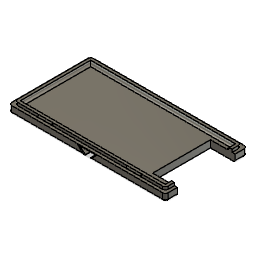
ROC_rev_C_screw_terminal_bottom (Autodesk Fusion 360 design; units mm, degrees)
Autodesk Fusion 360 part; units mm, degrees
sketch "Sketch13" plane through (0, 16, -2.5) normal (0, -1, 0) x (1, 0, 0)
  line L0 (26.9, -45.4) -> (26.9, -60.4)
  arc A0 (24.9, -62.4) -> (26.9, -60.4) centre (24.9, -60.4) ccw
  line L1 (24.9, -62.4) -> (-24.9, -62.4)
  arc A1 (-26.9, -60.4) -> (-24.9, -62.4) centre (-24.9, -60.4) ccw
  line L2 (-26.9, -60.4) -> (-26.9, -45.4)
  line L3 (-26.9, -45.4) -> (-26.9, -35.4)
  line L4 (-26.9, -35.4) -> (-26.9, 17.4)
  line L5 (-26.9, 17.4) -> (-26.9, 27.4)
  line L6 (-26.9, 27.4) -> (-26.9, 42.4)
  arc A2 (-24.9, 44.4) -> (-26.9, 42.4) centre (-24.9, 42.4) ccw
  line L7 (-24.9, 44.4) -> (24.9, 44.4)
  arc A3 (26.9, 42.4) -> (24.9, 44.4) centre (24.9, 42.4) ccw
  line L8 (26.9, 42.4) -> (26.9, 27.4)
  line L9 (26.9, 27.4) -> (26.9, 17.4)
  line L10 (26.9, 17.4) -> (26.9, -35.4)
  line L11 (26.9, -35.4) -> (26.9, -45.4)
  arc A4 (29, 44.5) -> (27, 46.5) centre (27, 44.5) ccw
  line L12 (27, 46.5) -> (-27, 46.5)
  arc A5 (-27, 46.5) -> (-29, 44.5) centre (-27, 44.5) ccw
  line L13 (-29, 44.5) -> (-29, -62.5)
  arc A6 (-29, -62.5) -> (-27, -64.5) centre (-27, -62.5) ccw
  line L14 (-27, -64.5) -> (27, -64.5)
  arc A7 (27, -64.5) -> (29, -62.5) centre (27, -62.5) ccw
  line L15 (29, -62.5) -> (29, 44.5)
  line L16 (-26.9, -35.4) -> (-29, -35.4)
  line L17 (-29, -35.4) -> (-29, -45.4)
  line L18 (-29, -45.4) -> (-26.9, -45.4)
  line L19 (-26.9, -45.4) -> (-26.9, -35.4)
  line L20 (-26.9, 27.4) -> (-29, 27.4)
  line L21 (-29, 27.4) -> (-29, 17.4)
  line L22 (-29, 17.4) -> (-26.9, 17.4)
  line L23 (-26.9, 17.4) -> (-26.9, 27.4)
  line L24 (26.9, 27.4) -> (29, 27.4)
  line L25 (29, 27.4) -> (29, 17.4)
  line L26 (29, 17.4) -> (26.9, 17.4)
  line L27 (26.9, 17.4) -> (26.9, 27.4)
  line L28 (26.9, -35.4) -> (29, -35.4)
  line L29 (29, -35.4) -> (29, -45.4)
  line L30 (29, -45.4) -> (26.9, -45.4)
  line L31 (26.9, -45.4) -> (26.9, -35.4)
  dimension "d1" = 10
  dimension "d2" = 2.1
  dimension "d3" = 10
  dimension "d4" = 10
  dimension "d5" = 10
  constraint horizontal L16
  constraint vertical L17
  constraint horizontal L18
  constraint vertical L19
  constraint coincident L3.end L4.start
  constraint horizontal L20
  constraint vertical L21
  constraint horizontal L22
  constraint vertical L23
  constraint coincident L5.end L6.start
  constraint horizontal L24
  constraint vertical L25
  constraint horizontal L26
  constraint vertical L27
  constraint coincident L8.end L9.start
  constraint horizontal L28
  constraint vertical L29
  constraint horizontal L30
  constraint vertical L31
  constraint coincident L10.end L11.start
  measures "d1" distance of L3.end L2.end
  measures "d2" distance of L5.end L20.end
  measures "d3" distance of L5.end L4.end
  measures "d4" distance of L8.end L9.end
  measures "d5" distance of L10.end L0.start
sketch "Sketch2" plane through (0, 0, 0) normal (0, 1, 0) x (1, 0, 0)
  line L0 (53.5, -29) -> (-53.5, -29)
  line L1 (-55.5, -27) -> (-55.5, 27)
  line L2 (-53.5, 29) -> (53.5, 29)
  line L3 (55.5, 27) -> (55.5, -27)
  line L4 (55.5, -29) -> (-55.5, 29) construction
  line L5 (-55.5, -29) -> (55.5, 29) construction
  arc A0 (-53.5, 29) -> (-55.5, 27) centre (-53.5, 27) ccw
  arc A1 (55.5, 27) -> (53.5, 29) centre (53.5, 27) ccw
  arc A2 (53.5, -29) -> (55.5, -27) centre (53.5, -27) ccw
  arc A3 (-55.5, -27) -> (-53.5, -29) centre (-53.5, -27) ccw
  dimension "d255" = 111
  dimension "d256" = 58
  dimension "d257" = 2
  dimension "d265" = 0
  dimension "d266" = 0
  dimension "d267" = 0
  dimension "d268" = 0
  dimension "d442" = 0
  dimension "d443" = 0
  dimension "d444" = 0
  dimension "d445" = 0
  dimension "d460" = 0
  dimension "d461" = 0
  dimension "d462" = 0
  dimension "d463" = 0
  constraint perpendicular L0 L1
  constraint parallel L0 L2
  constraint parallel L1 L3
  constraint horizontal L0
  constraint coincident L4 origin
  constraint coincident L5 origin
  constraint coincident L4.end L1
  constraint coincident L4.end L2
  constraint tangent L1 A0
  constraint tangent L2 A0
  constraint coincident L5.end L2
  constraint coincident L5.end L3
  constraint tangent L2 A1
  constraint tangent L3 A1
  constraint equal A0 A1
  constraint coincident L4.start L3
  constraint coincident L4.start L0
  constraint tangent L3 A2
  constraint tangent L0 A2
  constraint equal A0 A2
  constraint coincident L5.start L0
  constraint coincident L5.start L1
  constraint tangent L0 A3
  constraint tangent L1 A3
  constraint equal A0 A3
  measures "d255" distance of L4.end L5.end
  measures "d256" distance of L5.start L4.end
  measures "d257" radius of A0
extrude "Extrude1" add sketch "Sketch2" along normal blind 5
sketch "Sketch3" plane through (0, 5, 0) normal (0, 1, 0) x (-1, 0, 0)
  arc A0 (53.5, -29) -> (55.5, -27) centre (53.5, -27) ccw
  line L0 (55.5, -27) -> (55.5, 27)
  arc A1 (55.5, 27) -> (53.5, 29) centre (53.5, 27) ccw
  line L1 (53.5, 29) -> (-53.5, 29)
  arc A2 (-53.5, 29) -> (-55.5, 27) centre (-53.5, 27) ccw
  line L2 (-55.5, 27) -> (-55.5, -27)
  arc A3 (-55.5, -27) -> (-53.5, -29) centre (-53.5, -27) ccw
  line L3 (-53.5, -29) -> (53.5, -29)
  line L4 (53.4, -24.9) -> (53.4, 24.9)
  line L5 (51.4, 26.9) -> (-51.4, 26.9)
  line L6 (-53.4, 24.9) -> (-53.4, -24.9)
  line L7 (-51.4, -26.9) -> (51.4, -26.9)
  arc A4 (51.4, -26.9) -> (53.4, -24.9) centre (51.4, -24.9) ccw
  arc A5 (-53.4, -24.9) -> (-51.4, -26.9) centre (-51.4, -24.9) ccw
  arc A6 (-51.4, 26.9) -> (-53.4, 24.9) centre (-51.4, 24.9) ccw
  arc A7 (53.4, 24.9) -> (51.4, 26.9) centre (51.4, 24.9) ccw
  line L8 (-51.4, 24.9) -> (-51.4, -24.9)
  line L9 (-51.4, -24.9) -> (51.4, -24.9)
  line L10 (51.4, -24.9) -> (51.4, 24.9)
  line L11 (51.4, 24.9) -> (-51.4, 24.9)
  dimension "d261" = 2
  dimension "d262" = -2
  dimension "d277" = 2.1
  dimension "d278" = 2.1
  dimension "d279" = 2.1
  dimension "d280" = 2.1
  constraint parallel L0 L4
  constraint parallel L1 L5
  constraint parallel L2 L6
  constraint parallel L3 L7
  constraint tangent L4 A4
  constraint tangent L7 A4
  constraint tangent L7 A5
  constraint tangent L6 A5
  constraint equal A4 A5
  constraint tangent L5 A6
  constraint tangent L6 A6
  constraint equal A4 A6
  constraint tangent L5 A7
  constraint tangent L4 A7
  constraint equal A4 A7
  measures "d261" radius of A4
  measures "d277" distance of L3 L7
  measures "d278" distance of L0 L4
  measures "d279" distance of L1 L5
  measures "d280" distance of L2 L6
extrude "Extrude2" add sketch "Sketch3" along normal blind 2 contours L4 L5 L6 L7 A4 A5 A6 A7
sketch "Sketch4" plane through (0, 0, 26.9) normal (0, 0, 1) x (1, 0, 0)
  line L0 (-51.4, 5) -> (51.4, 5)
  line L1 (51.4, 5) -> (51.4, 7)
  line L2 (51.4, 7) -> (-51.4, 7)
  line L3 (-51.4, 7) -> (-51.4, 5)
  line L4 (36.4, 7) -> (26.4, 7)
  line L5 (26.4, 7) -> (26.4, 2)
  line L6 (26.4, 2) -> (36.4, 2)
  line L7 (36.4, 2) -> (36.4, 7)
  line L8 (-26.4, 7) -> (-36.4, 7)
  line L9 (-36.4, 7) -> (-36.4, 2)
  line L10 (-36.4, 2) -> (-26.4, 2)
  line L11 (-26.4, 2) -> (-26.4, 7)
  dimension "d289" = 10
  dimension "d290" = 10
  dimension "d291" = 15
  dimension "d292" = 15
  constraint horizontal L4
  constraint vertical L5
  constraint horizontal L6
  constraint vertical L7
  constraint coincident L2 L4.start
  constraint horizontal L8
  constraint vertical L9
  constraint horizontal L10
  constraint vertical L11
  constraint coincident L2 L8.start
  measures "d289" distance of L4.start L4.end
  measures "d290" distance of L8.start L8.end
  measures "d291" distance of L3 L9
  measures "d292" distance of L1 L7
extrude "Extrude3" add sketch "Sketch4" along normal blind 1 contours L0 L2 L8 L9 L11 | L0 L2 L4 L5 L7
sketch "Sketch5" plane through (-36.4, 0, 0) normal (-1, 0, 0) x (0, 0, 1)
  line L0 (26.9, 7) -> (26.9, 5)
  line L1 (26.9, 5) -> (27.9, 5)
  line L2 (27.9, 5) -> (27.9, 7)
  line L3 (27.9, 7) -> (26.9, 7)
  line L4 (26.9, 7) -> (27.9, 6)
  line L5 (26.9, 5) -> (27.9, 6)
  constraint coincident L0.start L3.end
  constraint midpoint L2 L4.end
  constraint coincident L0.end L1.start
extrude "Extrude4" cut sketch "Sketch5" against normal up to surface (72.8 mm away) contours L2 L3 L4 | L1 L2 L5
sketch "Sketch6" plane through (0, 0, -26.9) normal (0, 0, -1) x (-1, 0, 0)
  line L0 (-51.4, 5) -> (51.4, 5)
  line L1 (51.4, 5) -> (51.4, 7)
  line L2 (51.4, 7) -> (-51.4, 7)
  line L3 (-51.4, 7) -> (-51.4, 5)
  line L4 (36.4, 7) -> (26.4, 7)
  line L5 (26.4, 7) -> (26.4, 2)
  line L6 (26.4, 2) -> (36.4, 2)
  line L7 (36.4, 2) -> (36.4, 7)
  line L8 (-26.4, 7) -> (-36.4, 7)
  line L9 (-36.4, 7) -> (-36.4, 2)
  line L10 (-36.4, 2) -> (-26.4, 2)
  line L11 (-26.4, 2) -> (-26.4, 7)
  dimension "d297" = 10
  dimension "d298" = 10
  dimension "d299" = 15
  dimension "d300" = 15
  constraint horizontal L4
  constraint vertical L5
  constraint horizontal L6
  constraint vertical L7
  constraint coincident L2 L4.start
  constraint horizontal L8
  constraint vertical L9
  constraint horizontal L10
  constraint vertical L11
  constraint coincident L2 L8.start
  measures "d297" distance of L4.start L4.end
  measures "d298" distance of L8.start L8.end
  measures "d299" distance of L1 L7
  measures "d300" distance of L3 L9
extrude "Extrude5" add sketch "Sketch6" along normal blind 1 contours L0 L2 L8 L9 L11 | L0 L2 L4 L5 L7
sketch "Sketch7" plane through (36.4, 0, 0) normal (1, 0, 0) x (0, 0, -1)
  line L0 (26.9, 7) -> (26.9, 5)
  line L1 (26.9, 5) -> (27.9, 5)
  line L2 (27.9, 5) -> (27.9, 7)
  line L3 (27.9, 7) -> (26.9, 7)
  line L4 (26.9, 7) -> (27.9, 6)
  line L5 (27.9, 6) -> (26.9, 5)
  constraint coincident L0.start L3.end
  constraint midpoint L2 L4.end
  constraint coincident L0.end L1.start
extrude "Extrude6" cut sketch "Sketch7" against normal up to surface (72.8 mm away) contours L2 L3 L4 | L1 L2 L5
extrude "Extrude7" cut sketch "Sketch13" against normal blind 1 contours L11 L15 L28 L29 L30 L31 | L9 L15 L24 L25 L26 L27 | L3 L13 L16 L17 L18 L19 | L5 L13 L20 L21 L22 L23
chamfer "Chamfer1" [no effect]
fillet "Fillet1" radius 0.1 4 edges at (-31.4, 6, 27.9) (31.4, 6, 27.9) (-31.4, 6, -27.9) (31.4, 6, -27.9)
fillet "Fillet2" radius 1 8 edges at (-54.9142, 0, 28.4142) (-55.5, 0, 0) (-54.9142, 0, -28.4142) (0, 0, -29) (54.9142, 0, -28.4142) (55.5, 0, 0) (54.9142, 0, 28.4142) (0, 0, 29)
sketch "Sketch11" plane through (0, 5, 0) normal (0, 1, 0) x (-1, 0, 0)
  line L0 (-36.4, -26.9) -> (-51.4, -26.9)
  arc A0 (-53.4, -24.9) -> (-51.4, -26.9) centre (-51.4, -24.9) ccw
  line L1 (-53.4, -24.9) -> (-53.4, 24.9)
  arc A1 (-51.4, 26.9) -> (-53.4, 24.9) centre (-51.4, 24.9) ccw
  line L2 (-51.4, 26.9) -> (-36.4, 26.9)
  line L3 (53.5, 29) -> (-53.5, 29)
  arc A2 (-53.5, 29) -> (-55.5, 27) centre (-53.5, 27) ccw
  line L4 (-55.5, 27) -> (-55.5, -27)
  arc A3 (-55.5, -27) -> (-53.5, -29) centre (-53.5, -27) ccw
  line L5 (-53.5, -29) -> (53.5, -29)
  line L6 (-73, 20.5) -> (-38, 20.5)
  line L7 (-38, 20.5) -> (-38, -20.5)
  line L8 (-38, -20.5) -> (-73, -20.5)
  line L9 (-73, -20.5) -> (-73, 20.5)
  line L10 (-73, 20.5) -> (-38, -20.5) construction
  line L11 (-38, 20.5) -> (-73, -20.5) construction
  line L12 (-36.4, 26.9) -> (-26.4, 26.9)
  line L13 (-26.4, 26.9) -> (26.4, 26.9)
  line L14 (26.4, 26.9) -> (36.4, 26.9)
  line L15 (36.4, 26.9) -> (51.4, 26.9)
  arc A4 (53.4, 24.9) -> (51.4, 26.9) centre (51.4, 24.9) ccw
  line L16 (53.4, 24.9) -> (53.4, -24.9)
  arc A5 (51.4, -26.9) -> (53.4, -24.9) centre (51.4, -24.9) ccw
  line L17 (51.4, -26.9) -> (36.4, -26.9)
  line L18 (36.4, -26.9) -> (26.4, -26.9)
  line L19 (26.4, -26.9) -> (-26.4, -26.9)
  line L20 (-26.4, -26.9) -> (-36.4, -26.9)
  arc A6 (53.5, -29) -> (55.5, -27) centre (53.5, -27) ccw
  line L21 (55.5, -27) -> (55.5, 27)
  arc A7 (55.5, 27) -> (53.5, 29) centre (53.5, 27) ccw
  point P0 (-55.5, 0)
  dimension "d424" = 35
  dimension "d425" = 41
  constraint horizontal L6
  constraint perpendicular L6 L7
  constraint parallel L6 L8
  constraint parallel L7 L9
  constraint coincident L10 P0
  constraint coincident L11 P0
  constraint midpoint L4 P0
  measures "d424" distance of L6.start L6.end
  measures "d425" distance of L6.start L8.end
extrude "Extrude12" cut sketch "Sketch11" along normal mid plane 14 contours L1 L4 L6 L8 | L1 L6 L7 L8
sketch "Sketch12" plane through (0, 0, 29) normal (0, 0, 1) x (1, 0, 0)
  line L0 (-53.5, 1) -> (53.5, 1)
  line L1 (53.5, 1) -> (53.5, 5)
  line L2 (53.5, 5) -> (-53.5, 5)
  line L3 (-53.5, 5) -> (-53.5, 1)
  line L4 (-5.5, 4) -> (5.5, 4)
  line L5 (5.5, 4) -> (5.5, -4)
  line L6 (5.5, -4) -> (-5.5, -4)
  line L7 (-5.5, -4) -> (-5.5, 4)
  line L8 (-5.5, 4) -> (5.5, -4) construction
  line L9 (5.5, 4) -> (-5.5, -4) construction
  line L10 (5.5, 0) -> (-5.5, 0)
  line L11 (5.5, 4) -> (11.438, 4) construction
  line L12 (-5.5, 4) -> (-1.5, 0)
  line L13 (-5.5, 4) -> (1, 4) construction
  line L14 (5.5, 4) -> (1.5, 0)
  line L15 (0.8684, -0.6316) -> (0.7116, -0.7884)
  dimension "d428" = 11
  dimension "d429" = 8
  dimension "d432" = 135
  dimension "d433" = 45
  constraint horizontal L4
  constraint perpendicular L4 L5
  constraint parallel L4 L6
  constraint parallel L5 L7
  constraint coincident L8 origin
  constraint coincident L9 origin
  constraint midpoint L5 L10.start
  constraint midpoint L7 L10.end
  constraint horizontal L11
  constraint horizontal L13
  constraint coincident L10 L14.end
  constraint coincident L8 L15.start
  constraint collinear L14 L15
  constraint coincident L10 L12.end
  measures "d428" distance of L5.end L6.end
  measures "d429" distance of L4.end L5.end
  measures "d432" angle of L11 L14
  measures "d433" angle of L12 L13
extrude "Extrude13" cut sketch "Sketch12" against normal up to surface (58 mm away) contours L0 L4 L12 L14 | L0 L10 L12 L14
chamfer "Chamfer2" distance 0.5 angle 45 12 edges at (-4, 2.5, -29) (-1.7929, 0.2929, -28.7071) (-1.5, 0, 0) (4, 2.5, 29) (1.7929, 0.2929, 28.7071) (1.5, 0, 0) (1.7929, 0.2929, -28.7071) (4, 2.5, -29) (-4, 2.5, 29) (-1.7929, 0.2929, 28.7071) (0, 4, 29) (0, 4, -29)
fillet "Fillet3" radius 2 5 edges at (0, 5, 24.9) (-51.4, 5, 0) (0, 5, -24.9) (51.4, 5, -22.7) (51.4, 5, 22.7)
